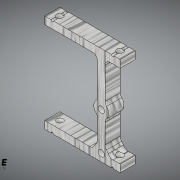
# Autodesk Inventor part: ウイング土台
Saved by Autodesk Inventor 2019 (Build 230136000, 136)
## iProperties
Created: 2019-11-29
Part Number: ウイング土台
Material: アルミニウム 7075
Document SubType Name: Modeling
Designer: tanjihayato
Density: 2.81 g/cm^3
Appearance: サテン - ブラシ仕上げ 重厚
Author: tanjihayato
Autodesk Inventor part; units mm, degrees
note: some values were not read from the file. Chosen so that the rebuilt part matches the saved one: sketch regions of "押し出し1".
ref_plane "YZ Plane" through (0, 0, 0) normal (1, 0, 0) x (0, 1, 0)
ref_plane "XZ Plane" through (0, 0, 0) normal (0, 1, 0) x (-1, 0, 0)
ref_plane "XY Plane" through (0, 0, 0) normal (0, 0, 1) x (1, 0, 0)
sketch "スケッチ1" plane through (0, 0, 0) normal (0, 0, 1) x (1, 0, 0)
  line L0 (0, 0) -> (30, 0)
  line L1 (30, 0) -> (30, -3)
  line L2 (30, -3) -> (24, -3)
  line L3 (24, -3) -> (24, -36)
  line L4 (24, -36) -> (30, -36)
  line L5 (30, -36) -> (30, -39)
  line L6 (30, -39) -> (0, -39)
  line L7 (0, -39) -> (0, -36)
  line L8 (0, -36) -> (21, -36)
  line L9 (21, -36) -> (21, -3)
  line L10 (21, -3) -> (0, -3)
  line L11 (0, -3) -> (0, 0)
  circle A0 centre (22.5, -36) radius 3
  circle A1 centre (22.5, -21) radius 3
  circle A2 centre (22.5, -21) radius 1.25
  circle A3 centre (22.5, -36) radius 1.25
  circle A4 centre (3, 0) radius 0.5
  circle A5 centre (27, 0) radius 0.5
  circle A6 centre (27, -39) radius 0.5
  circle A7 centre (3, -39) radius 0.5
  dimension "d0" = 30
  dimension "d1" = 3
  dimension "d2" = 3
  dimension "d3" = 3
  dimension "d4" = 39
  dimension "d5" = 6
  dimension "d6" = 6
  dimension "d7" = 6
  dimension "d8" = 15
  dimension "d9" = 1.5
  dimension "d10" = 3
  dimension "d11" = 2.5
  dimension "d12" = 2.5
  dimension "d14" = 1
  dimension "d15" = 1
  dimension "d16" = 1
  dimension "d17" = 1
  dimension "d18" = 3
  dimension "d19" = 3
  dimension "d20" = 3
  dimension "d21" = 3
  constraints: 24 end point, 11 point on line, 8 centre point, 8 perpendicular, 2 coincident, 1 horizontal, 1 vertical alignment
  measures "d0" distance of L0.start L0.end
  measures "d1" distance of L0.end L1.end
  measures "d2" distance of L4.end L5.end
  measures "d3" distance between parallel lines of L3 L9
  measures "d4" distance between parallel lines of L6 L0
  measures "d5" distance between parallel lines of L3 L1
  measures "d6" diameter of A0
  measures "d7" diameter of A1
  measures "d8" distance of A0.centre A1.centre
  measures "d9" distance from line of L3 A1.centre
  measures "d10" distance from line of L6 A0.centre
  measures "d11" diameter of A2
  measures "d12" diameter of A3
  measures "d14" diameter of A4
  measures "d15" diameter of A5
  measures "d16" diameter of A6
  measures "d17" diameter of A7
  measures "d18" distance from line of L11 A4.centre
  measures "d19" distance from line of L7 A7.centre
  measures "d20" distance from line of L5 A6.centre
  measures "d21" distance from line of L1 A5.centre
extrude "押し出し1" add sketch "スケッチ1" along normal blind 6 contours A5 L0 | L0 L1 L2 L3 A1 L9 L10 L11 A4 A5 | A4 L0 | A1 L3 | L3 A1 L9 | L3 A0 L9 A1 | L9 A1 | A0 L4 L3 | L3 L4 A0 L8 L9 | L4 L5 L6 A6 A0 | L9 L8 A0 | L6 A7 L7 L8 A0 | A6 L6 | L6 A7 picked at (26.9053, -0.1372) picked at (2.8382, -0.0399) picked at (27.0201, -38.8345) picked at (3.0201, -38.8345)
extrude "押し出し2" cut sketch "スケッチ1" along normal blind 6 contours A5 L0 | L0 A5 | A4 L0 | L0 A4 | A6 L6 | L6 A6 | A7 L6 | L6 A7
fillet "フィレット1" radius 2 10 edges at (24, -3, 3) (21, -3, 3) (24, -23.5981, 3) (24, -18.4019, 3) (21, -23.5981, 3) (21, -18.4019, 3) (24, -33.4019, 3) (21, -33.4019, 3) (19.5, -36, 3) (25.5, -36, 3)
sketch "スケッチ2" plane through (3.5, -39, 0) normal (0, -1, 0) x (1, 0, 0)
  line L0 (0, 6) -> (0, 0) projected
  line L1 (-1, 6) -> (0, 6) projected
  line L2 (-1, 0) -> (-1, 6) projected
  line L3 (0, 0) -> (-1, 0) projected
  line L4 (24, 6) -> (24, 0) projected
  line L5 (23, 6) -> (24, 6) projected
  line L6 (23, 0) -> (23, 6) projected
  line L7 (24, 0) -> (23, 0) projected
  circle A0 centre (-0.5, 3) radius 1.25
  circle A1 centre (23.5, 3) radius 1.25
  point P0 (-3.5, 0)
  dimension "d27" = 2.5
  dimension "d28" = 2.5
  dimension "d29" = 3
  dimension "d30" = 0.5
  dimension "d31" = 3
  dimension "d32" = 0.5
  constraints: 2 centre point
  measures "d27" diameter of A0
  measures "d28" diameter of A1
  measures "d29" distance from line of A1.centre L5
  measures "d30" distance from line of A1.centre L4
  measures "d31" distance from line of A0.centre L3
  measures "d32" distance from line of A0.centre L0
extrude "押し出し3" cut sketch "スケッチ2" against normal blind 40 contours A0 L0 | L0 A0 L2 | L2 A0 | A1 L4 | L4 A1 L6 | L6 A1
